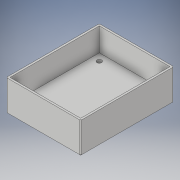
# Autodesk Inventor part: Enclosure Rev A
Saved by Autodesk Inventor 2017 (Build 210142000, 142)
## iProperties
Created: 2016-04-29
Part Number: Enclosure Rev A
Material: Generic
Document SubType Name: Modeling
Designer: Casey Laptop
Density: 1 g/cm^3
Appearance: Default
Author: Casey Laptop
Autodesk Inventor part; units mm, degrees
ref_plane "YZ Plane" through (0, 0, 0) normal (1, 0, 0) x (0, 1, 0)
ref_plane "XZ Plane" through (0, 0, 0) normal (0, 1, 0) x (-1, 0, 0)
ref_plane "XY Plane" through (0, 0, 0) normal (0, 0, 1) x (1, 0, 0)
sketch "Sketch1" plane through (0, 0, 0) normal (0, 1, 0) x (-1, 0, 0)
  line L0 (30.48, 38.1) -> (-30.48, 38.1)
  line L1 (-30.48, 38.1) -> (-30.48, -38.1)
  line L2 (-30.48, -38.1) -> (30.48, -38.1)
  line L3 (30.48, -38.1) -> (30.48, 38.1)
  point P0 (0, 0)
  dimension "d0" = 76.2
  dimension "d1" = 60.96
  dimension "d2" = 38.1
  dimension "d3" = 30.48
  constraints: 8 end point, 2 parallel, 1 horizontal, 1 perpendicular
  measures "d0" distance between parallel lines of L2 L0
  measures "d1" distance of L1.end L2.end
  measures "d2" distance from line of L2 point (0, 0)
  measures "d3" distance from line of point (0, 0) L1
extrude "Extrusion1" add sketch "Sketch1" along normal blind 25.4
sketch "Sketch2" plane through (0, 25.4, 0) normal (0, 1, 0) x (1, 0, 0)
  line L0 (-28.8925, 36.5125) -> (28.8925, 36.5125)
  line L1 (28.8925, 36.5125) -> (28.8925, -36.5125)
  line L2 (28.8925, -36.5125) -> (-28.8925, -36.5125)
  line L3 (-28.8925, -36.5125) -> (-28.8925, 36.5125)
  point P0 (0, 0)
  dimension "d6" = 73.025
  dimension "d7" = 57.785
  dimension "d8" = 36.5125
  dimension "d9" = 28.8925
  constraints: 8 end point, 2 parallel, 1 horizontal, 1 perpendicular
  measures "d6" distance of L2.end L0.start
  measures "d7" distance of L0.start L0.end
  measures "d8" distance from line of point (0, 0) L0
  measures "d9" distance from line of point (0, 0) L1
extrude "Extrusion2" cut sketch "Sketch2" against normal blind 19.05
chamfer "Chamfer1" distance 0.7937 angle 45 8 edges at (0, 0, 38.1) (30.48, 0, 0) (0, 0, -38.1) (-30.48, 0, 0) (30.48, 12.7, 38.1) (-30.48, 12.7, 38.1) (30.48, 12.7, -38.1) (-30.48, 12.7, -38.1)
sketch "Sketch3" plane through (0, 6.35, 0) normal (0, 1, 0) x (1, 0, 0)
  circle A0 centre (-22.86, 30.48) radius 1.9304
  circle A1 centre (22.86, 30.48) radius 1.9304
  circle A2 centre (-22.86, -30.48) radius 1.9304
  circle A3 centre (22.86, -30.48) radius 1.9304
  line L0 (-28.8925, -36.5125) -> (-28.8925, 36.5125) projected
  line L1 (-28.8925, 36.5125) -> (28.8925, 36.5125) projected
  line L2 (0, 0) -> (0, 32.9664)
  line L3 (0, 0) -> (-24.0434, 0)
  line L4 (0, 0) -> (25.6064, 0)
  line L5 (0, 0) -> (0, -31.6413)
  dimension "d15" = 3.8608
  dimension "d16" = 3.8608
  dimension "d17" = 3.8608
  dimension "d18" = 3.8608
  dimension "d21" = 30.48
  dimension "d22" = 22.86
  dimension "d23" = 22.86
  dimension "d24" = 30.48
  dimension "d25" = 22.86
  dimension "d26" = 30.48
  dimension "d27" = 22.86
  dimension "d28" = 30.48
  constraints: 8 end point, 4 centre point, 2 horizontal, 2 vertical
  measures "d15" diameter of A0
  measures "d16" diameter of A1
  measures "d17" diameter of A2
  measures "d18" diameter of A3
  measures "d21" distance from line of L3 A0.centre
  measures "d22" distance from line of L2 A0.centre
  measures "d23" distance from line of L2 A1.centre
  measures "d24" distance from line of L4 A1.centre
  measures "d25" distance from line of L5 A2.centre
  measures "d26" distance from line of L3 A2.centre
  measures "d27" distance from line of L5 A3.centre
  measures "d28" distance from line of L4 A3.centre
extrude "Extrusion3" cut sketch "Sketch3" against normal blind 6.35
sketch "Sketch4" plane through (0, 0, 0) normal (0, -1, 0) x (1, 0, 0)
  circle A0 centre (-22.86, 30.48) radius 5.08
  line L0 (0, 0) -> (-26.2361, 0)
  line L1 (-26.2361, 0) -> (0, 0)
  line L2 (0, 0) -> (0, 35.0708)
  line L3 (0, 0) -> (27.0223, 0)
  line L4 (0, 0) -> (0, -33.193)
  circle A1 centre (22.86, 30.48) radius 5.08
  circle A2 centre (-22.86, -30.48) radius 5.08
  circle A3 centre (22.86, -30.48) radius 1.9304 projected
  circle A4 centre (22.86, -30.48) radius 5.08
  dimension "d31" = 10.16
  dimension "d32" = 22.86
  dimension "d33" = 30.48
  dimension "d34" = 10.16
  dimension "d35" = 22.86
  dimension "d36" = 30.48
  dimension "d37" = 10.16
  dimension "d38" = 10.16
  dimension "d39" = 30.48
  dimension "d40" = 22.86
  constraints: 10 end point, 4 centre point, 2 horizontal, 2 vertical, 1 coincident, 1 collinear
  measures "d31" diameter of A0
  measures "d32" distance from line of L2 A0.centre
  measures "d33" distance from line of L0 A0.centre
  measures "d34" diameter of A1
  measures "d35" distance from line of L2 A1.centre
  measures "d36" distance from line of L3 A1.centre
  measures "d37" diameter of A4
  measures "d38" diameter of A2
  measures "d39" distance from line of L0 A2.centre
  measures "d40" distance from line of L4 A2.centre
extrude "Extrusion4" cut sketch "Sketch4" against normal blind 3.175
body "Solid1"
